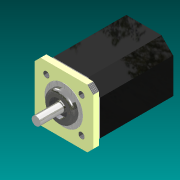
# Autodesk Inventor part: 电机
Saved by Autodesk Inventor 2021 (Build 250183000, 183)
## iProperties
Created: 2024-06-10
Part Number: 电机
Material: 常规
Document SubType Name: Modeling
Designer: 86155
Density: 1 g/cm^3
Appearance: 默认
Author: 86155
Autodesk Inventor part; units mm, degrees
ref_plane "YZ Plane" through (0, 0, 0) normal (1, 0, 0) x (0, 1, 0)
ref_plane "XZ Plane" through (0, 0, 0) normal (0, 1, 0) x (-1, 0, 0)
ref_plane "XY Plane" through (0, 0, 0) normal (0, 0, 1) x (1, 0, 0)
sketch "草图1" plane through (0, 0, 0) normal (0, 0, 1) x (1, 0, 0)
  line L0 (-100, 100) -> (100, 100)
  line L1 (100, 100) -> (100, -100)
  line L2 (100, -100) -> (-100, -100)
  line L3 (-100, -100) -> (-100, 100)
  line L4 (-100, 100) -> (100, -100) construction
  line L5 (100, 100) -> (-100, -100) construction
  point P0 (0, 0)
  dimension "d0" = 200
  dimension "d1" = 200
  constraints: 12 end point, 2 midpoint, 2 parallel, 1 horizontal, 1 perpendicular
  measures "d0" distance of L1.end L2.end
  measures "d1" distance of L0.end L1.end
extrude "拉伸1" add sketch "草图1" along normal blind 250
sketch "草图3" plane through (0, 0, 250) normal (0, 0, 1) x (1, 0, 0)
  line L0 (-90, 90) -> (90, 90)
  line L1 (90, 90) -> (90, -90)
  line L2 (90, -90) -> (-90, -90)
  line L3 (-90, -90) -> (-90, 90)
  line L4 (-90, 90) -> (90, -90) construction
  line L5 (90, 90) -> (-90, -90) construction
  point P0 (0, 0)
  dimension "d6" = 180
  dimension "d7" = 180
  constraints: 12 end point, 2 midpoint, 2 parallel, 1 horizontal, 1 perpendicular
  measures "d6" distance of L1.end L2.end
  measures "d7" distance of L0.end L1.end
extrude "拉伸2" add sketch "草图3" along normal blind 3
chamfer "倒角1" distance 40 angle 45 4 edges at (100, 100, 125) (-100, -100, 125) (100, -100, 125) (-100, 100, 125)
sketch "草图4" plane through (0, 0, 253) normal (0, 0, 1) x (1, 0, 0)
  line L0 (-100, 100) -> (100, 100)
  line L1 (100, 100) -> (100, -100)
  line L2 (100, -100) -> (-100, -100)
  line L3 (-100, -100) -> (-100, 100)
  line L4 (-100, 100) -> (100, -100) construction
  line L5 (100, 100) -> (-100, -100) construction
  point P0 (0, 0)
  dimension "d10" = 200
  dimension "d11" = 200
  constraints: 12 end point, 2 midpoint, 2 parallel, 1 horizontal, 1 perpendicular
  measures "d10" distance of L1.end L2.end
  measures "d11" distance of L0.end L1.end
extrude "拉伸3" add sketch "草图4" along normal blind 20
sketch "草图5" plane through (0, 0, 273) normal (0, 0, 1) x (1, 0, 0)
  circle A0 centre (0, 0) radius 50
  dimension "d17" = 100
  constraints: 1 centre point, 1 coincident
  measures "d17" diameter of A0
extrude "拉伸4" add sketch "草图5" along normal blind 20
fillet "圆角1" radius 10 1 edges at (-50, 0, 293)
sketch "草图6" plane through (0, 0, 273) normal (0, 0, 1) x (1, 0, 0)
  circle A0 centre (0, 0) radius 65
  dimension "d21" = 130
  constraints: 1 centre point, 1 coincident
  measures "d21" diameter of A0
extrude "拉伸5" add sketch "草图6" along normal blind 1
sketch "草图7" plane through (0, 0, 293) normal (0, 0, 1) x (1, 0, 0)
  circle A0 centre (0, 0) radius 30
  dimension "d24" = 60
  constraints: 1 centre point, 1 coincident
  measures "d24" diameter of A0
extrude "拉伸6" cut sketch "草图7" against normal blind 15
sketch "草图8" plane through (0, 0, 278) normal (0, 0, 1) x (1, 0, 0)
  circle A0 centre (0, 0) radius 17.5
  dimension "d27" = 35
  constraints: 1 centre point, 1 coincident
  measures "d27" diameter of A0
extrude "拉伸7" add sketch "草图8" along normal blind 10
sketch "草图9" plane through (0, 0, 288) normal (0, 0, 1) x (1, 0, 0)
  circle A0 centre (0, 0) radius 15
  dimension "d30" = 30
  constraints: 1 centre point, 1 coincident
  measures "d30" diameter of A0
extrude "拉伸8" add sketch "草图9" along normal blind 80
sketch "草图10" plane through (0, 0, 273) normal (0, 0, 1) x (1, 0, 0)
  point P0 (0, 0)
  point P1 (-60, 60)
  point P2 (60, 60)
  point P3 (60, -60)
  point P4 (-60, -60)
  dimension "d33" = 60
  dimension "d34" = 60
  dimension "d37" = 360
  constraints: 5 other
  measures "d33" horizontal distance of point (0, 0) point (-60, 60)
  measures "d34" horizontal distance of point (0, 0) point (-60, 60)
hole "孔1" at (-60, 60, 273) at (60, 60, 273) at (60, -60, 273) at (-60, -60, 273) direction (0, 0, -1) diameter 20.752 depth 61.1 tip angle 118 thread size "M24x3" designation "M24" class "6H" standard "GB Metric profile"
chamfer "倒角2" distance 20 angle 45 4 edges at (-100, -100, 263) (100, -100, 263) (100, 100, 263) (-100, 100, 263)
scale "缩放比例1" factors (0.4, 0.4, 0.4) then translate (0, 0, 0) bodies 1
